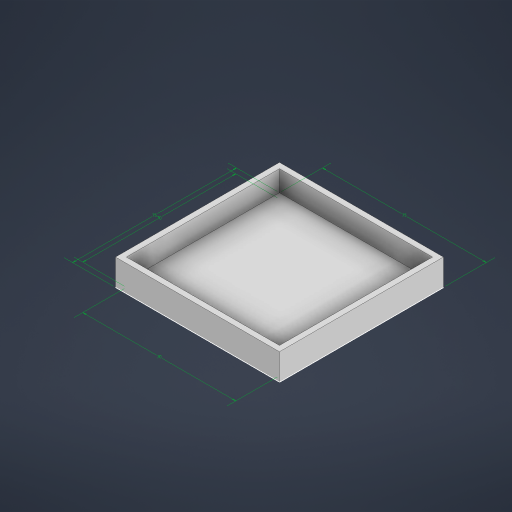
# Autodesk Inventor part: boxCap
Saved by Autodesk Inventor 2023 (Build 270158000, 158)
## iProperties
Created: 2022-09-23
Part Number: boxCap
Material: Generic
Document SubType Name: Modeling
Designer: Vlasciar
Density: 1 g/cm^3
Appearance: Default
Author: Vlasciar
Autodesk Inventor part; units mm, degrees
ref_plane "YZ Plane" through (0, 0, 0) normal (1, 0, 0) x (0, 1, 0)
ref_plane "XZ Plane" through (0, 0, 0) normal (0, 1, 0) x (-1, 0, 0)
ref_plane "XY Plane" through (0, 0, 0) normal (0, 0, 1) x (1, 0, 0)
sketch "Sketch1" plane through (0, 0, 0) normal (0, 1, 0) x (-1, 0, 0)
  line L0 (-37.5, 37.5) -> (37.5, 37.5)
  line L1 (37.5, 37.5) -> (37.5, -37.5)
  line L2 (37.5, -37.5) -> (-37.5, -37.5)
  line L3 (-37.5, -37.5) -> (-37.5, 37.5)
  line L4 (-37.5, 37.5) -> (37.5, -37.5) construction
  line L5 (37.5, 37.5) -> (-37.5, -37.5) construction
  line L6 (-35, -35) -> (35, -35)
  line L7 (35, -35) -> (35, 35)
  line L8 (35, 35) -> (-35, 35)
  line L9 (-35, 35) -> (-35, -35)
  line L10 (-35, -35) -> (35, 35) construction
  line L11 (35, -35) -> (-35, 35) construction
  point P0 (0, 0)
  dimension "d0" = 75
  dimension "d1" = 75
  dimension "d2" = 70
  dimension "d3" = 70
  constraints: 24 end point, 4 midpoint, 4 parallel, 2 horizontal, 2 perpendicular
  measures "d0" distance of L1.end L2.end
  measures "d1" distance of L0.end L1.end
  measures "d2" distance of L8.end L7.end
  measures "d3" distance of L7.end L6.end
extrude "Extrusion1" add sketch "Sketch1" along normal blind 12
extrude "Extrusion2" add sketch "Sketch1" along normal blind 2.5 contours L9 L8 L7 L6
body "Solid1"
